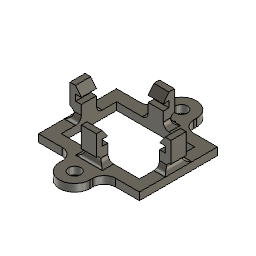
5v Reg bracket (Autodesk Fusion 360 design; units mm, degrees)
part number: 2026-03-18-18-39-53-770
Autodesk Fusion 360 part; units mm, degrees
sketch "Sketch1" plane through (0, 0, 0) normal (0, 0, 1) x (1, 0, 0)
  line L0 (-11.75, 8.75) -> (11.75, 8.75)
  line L1 (11.75, 8.75) -> (11.75, -8.75)
  line L2 (11.75, -8.75) -> (-11.75, -8.75)
  line L3 (-11.75, -8.75) -> (-11.75, 8.75)
  line L4 (-13.25, 10.25) -> (13.25, 10.25)
  line L5 (13.25, 10.25) -> (13.25, -10.25)
  line L6 (13.25, -10.25) -> (-13.25, -10.25)
  line L7 (-13.25, -10.25) -> (-13.25, 10.25)
  line L8 (-13.25, 10.25) -> (13.25, -10.25) construction
  line L9 (-13.25, -10.25) -> (13.25, 10.25) construction
  circle A0 centre (0, 14) radius 1.6
  circle A1 centre (0, -14) radius 1.6
  circle A2 centre (0, 14) radius 4
  circle A3 centre (0, -14) radius 4
  line L10 (-4, 14) -> (-4, 10.25)
  line L11 (4, 14) -> (4, 10.25)
  line L12 (4, -14) -> (4, -10.25)
  line L13 (-4, -14) -> (-4, -10.25)
  line L14 (-10.25, 7.25) -> (10.25, 7.25)
  line L15 (10.25, 7.25) -> (10.25, -7.25)
  line L16 (10.25, -7.25) -> (-10.25, -7.25)
  line L17 (-10.25, -7.25) -> (-10.25, 7.25)
  line L18 (-10.25, 7.25) -> (10.25, -7.25) construction
  line L19 (10.25, 7.25) -> (-10.25, -7.25) construction
  line L20 (-13.25, -2) -> (-10.25, -2)
  line L21 (-10.25, -2) -> (-10.25, 2)
  line L22 (-10.25, 2) -> (-13.25, 2)
  line L23 (-13.25, 2) -> (-13.25, -2)
  line L24 (-13.25, 2) -> (-10.25, -2) construction
  line L25 (13.25, -2) -> (10.25, -2)
  line L26 (10.25, -2) -> (10.25, 2)
  line L27 (10.25, 2) -> (13.25, 2)
  line L28 (13.25, 2) -> (13.25, -2)
  line L29 (-2, 7.25) -> (2, 7.25)
  line L30 (2, 7.25) -> (2, 10.75)
  line L31 (-2, 10.75) -> (-2, 7.25)
  line L32 (-2, -10.25) -> (2, -10.25)
  line L33 (2, -10.25) -> (2, -7.25)
  line L34 (2, -7.25) -> (-2, -7.25)
  line L35 (-2, -7.25) -> (-2, -10.25)
  point P0 (0, 8.75)
  point P1 (-11.75, 0)
  dimension "boardL" = 23.5
  dimension "boardW" = 17.5
  dimension "d3" = 0
  dimension "d4" = 0
  dimension "d5" = 26.5
  dimension "d6" = 20.5
  dimension "dScrew" = 3.2
  dimension "d8" = 3.2
  dimension "screwOffset" = 14
  dimension "d10" = 14
  dimension "dScrewBase" = 8
  dimension "d12" = 8
  dimension "d27" = 14.5
  dimension "d28" = 20.5
  dimension "smallSideSupportW" = 4
  dimension "d38" = 2
  dimension "d39" = 4
  dimension "d40" = 2
  dimension "largeSideSupportW" = 4
  dimension "d42" = 2
  dimension "d43" = 4
  dimension "d44" = 2
  constraint horizontal L0
  constraint vertical L1
  constraint horizontal L2
  constraint vertical L3
  constraint midpoint L0 P0
  constraint midpoint L3 P1
  constraint horizontal L4
  constraint vertical L5
  constraint horizontal L6
  constraint vertical L7
  constraint midpoint origin L9
  constraint concentric A0 A2
  constraint concentric A1 A3
  constraint coincident A2 L10.start
  constraint coincident L4 L10.end
  constraint perpendicular L4 L10
  constraint coincident A2 L11.start
  constraint coincident L4 L11.end
  constraint perpendicular L4 L11
  constraint coincident A3 L12.start
  constraint coincident L6 L12.end
  constraint perpendicular L6 L12
  constraint coincident A3 L13.start
  constraint coincident L6 L13.end
  constraint perpendicular L6 L13
  constraint horizontal L14
  constraint vertical L15
  constraint horizontal L16
  constraint vertical L17
  constraint midpoint origin L19
  constraint horizontal L20
  constraint vertical L21
  constraint horizontal L22
  constraint vertical L23
  constraint coincident L7 L20.start
  constraint horizontal L25
  constraint vertical L26
  constraint horizontal L27
  constraint vertical L28
  constraint coincident L5 L25.start
  constraint horizontal L29
  constraint vertical L30
  constraint vertical L31
  constraint coincident L14 L29.start
  constraint horizontal L32
  constraint vertical L33
  constraint horizontal L34
  constraint vertical L35
  constraint coincident L6 L32.start
  constraint coincident L17 L21.end
  constraint coincident L15 L26.end
  constraint coincident L16 L34.end
  measures "boardL" distance of L0.start L0.end
  measures "boardW" distance of L0.start L2.end
  measures "d3" horizontal distance of origin P0
  measures "d4" vertical distance of origin P1
  measures "d5" distance of L4.start L4.end
  measures "d6" distance of L4.start L6.end
  measures "dScrew" diameter of A0
  measures "d8" diameter of A1
  measures "screwOffset" distance of origin A0.centre
  measures "d10" distance of origin A1.centre
  measures "dScrewBase" diameter of A2
  measures "d12" diameter of A3
  measures "d27" distance of L14.start L16.end
  measures "d28" distance of L14.start L14.end
  measures "smallSideSupportW" distance of L20.start L22.end
  measures "d38" vertical distance of origin L22.end
  measures "d39" distance of L25.start L27.end
  measures "d40" vertical distance of origin L25.start
  measures "largeSideSupportW" distance of L29.start L29.end
  measures "d42" horizontal distance of origin L30.end
  measures "d43" distance of L32.start L32.end
  measures "d44" horizontal distance of origin L34.end
extrude "Extrude7" add sketch "Sketch1" along normal blind 2 contours L0 L3 L4 L7 L22 L31 | L0 L3 L14 L17 L22 L31 | L0 L4 A2 L30 L31 | L0 L14 L29 L30 L31 | L3 L17 L20 L21 L22 | L3 L7 L20 L22 L23 | L0 L1 L4 L5 L27 L30 | L0 L1 L14 L15 L27 L30 | L4 A2 L10 L31 | L2 L3 L16 L17 L20 L35 | L2 L3 L6 L7 L20 L35 | L4 A2 L11 L30 | L4 A2 | L4 A2 | L1 L5 L25 L27 L28 | L1 L15 L25 L26 L27 | L2 L16 L33 L34 L35 | L2 L6 A3 L32 L33 L35 | L1 L2 L5 L6 L25 L33 | L1 L2 L15 L16 L25 L33 | L6 A3 L13 L32 | L6 A3 L12 L32 | L6 A3 L32 | L6 A3 L32 makes body 1
extrude "Extrude10" add sketch "Sketch1" along normal blind 9.6 separate body contours L0 L4 A2 L30 L31 | L0 L14 L29 L30 L31 | L3 L17 L20 L21 L22 | L3 L7 L20 L22 L23 | L4 A2 | L1 L5 L25 L27 L28 | L1 L15 L25 L26 L27 | L2 L16 L33 L34 L35 | L2 L6 A3 L32 L33 L35 | L6 A3 L32 picked at (0.2822, 10.1969) picked at (0.2765, -10.1169) makes body 2 at (0.6667, -10.25, 6.4) makes body 3 at (-10.25, -0.6667, 3.2) makes body 4 at (10.25, 0.6667, 3.2) makes body 5 at (-0.6667, 10.25, 3.2)
extrude "Extrude11" add sketch "Sketch1" along normal blind 1.6 from surface at 6 separate body contours L0 L3 L14 L17 L22 L31 | L0 L14 L29 L30 L31 | L3 L17 L20 L21 L22 | L0 L1 L14 L15 L27 L30 | L14 L15 L16 L17 L21 L26 L29 L34 | L2 L3 L16 L17 L20 L35 | L1 L15 L25 L26 L27 | L2 L16 L33 L34 L35 | L1 L2 L15 L16 L25 L33 makes body 6
combine "Combine2" operation cut target body 2 tool bodies 6 keep tools
combine "Combine3" operation cut target body 3 tool bodies 6 keep tools
combine "Combine4" operation cut target body 5 tool bodies 6 keep tools
combine "Combine5" operation cut target body 4 tool bodies 6
chamfer "Chamfer1" distance 1.5 distance2 2 4 edges at (-10.25, 0, 9.6) (10.25, 0, 9.6) (0, -7.25, 9.6) (0, 7.25, 9.6) measured on face at (-12.25, -0.6667, 9.6) measured on face at (11.25, -0.6667, 9.6) measured on face at (0.6667, -9.25, 9.6) measured on face at (-0.6667, 9.25, 9.6) on bodies 2 3 4 5
fillet "Fillet5" radius 3 6 edges at (-2, 10.25, 1) (-4, 10.25, 1) (4, 10.25, 1) (2, 10.25, 1) (4, -10.25, 1) (-4, -10.25, 1) on bodies 1
combine "Combine6" operation add target body 3 tool bodies 1 5 4 2
fillet "Fillet6" radius 1.5 8 edges at (-11.75, -2, 2) (-2, -8.75, 2) (11.75, -2, 2) (-2, 8.75, 2) (2, -8.75, 2) (2, 8.75, 2) (11.75, 2, 2) (-11.75, 2, 2) on bodies 3
pipe "Pipe1" add diameter 2.2 path "Sketch1" along L5 L6 L7 L4 separate body makes body 7
move_body "Move1" bodies 7 to x (1, 0, 0) y (0, 1, 0) z (0, 0, 1) at (0, 0, 3.1)
combine "Combine7" operation cut target body 3 tool bodies 7
equation "d5 = boardL + 3 mm"
equation "d6 = boardW + 3 mm"
equation "d8 = dScrew"
equation "d10 = screwOffset"
equation "d12 = dScrewBase"
equation "d27 = boardW - 3 mm"
equation "d28 = boardL - 3 mm"
equation "d38 = smallSideSupportW / 2"
equation "d39 = smallSideSupportW"
equation "d40 = smallSideSupportW / 2"
equation "d42 = largeSideSupportW / 2"
equation "d43 = largeSideSupportW"
equation "d44 = largeSideSupportW / 2"
equation "baseHeight = basePlateH"
equation "boardH = 1.6 mm"
equation "gripHeight = 2 mm"
equation "boardZOffset = 6 mm"
equation "d56 = boardZOffset + boardH + gripHeight"
equation "d58 = boardZOffset"
equation "d59 = boardH"
equation "d69 = easeRingDiameter"
equation "d73 = basePlateH + easeRingDiameter / 2"
equation "easeRingDiameter = 2.2 mm"
equation "basePlateH = 2 mm"
